Metal Shelf Foot (Autodesk Fusion 360 design; units mm, degrees)
Autodesk Fusion 360 part; units mm, degrees
sketch "Sketch1" plane through (0, 0, 0) normal (0, 0, 1) x (1, 0, 0)
  line L0 (0, 0) -> (46, 0)
  line L1 (46, 0) -> (46, 32)
  line L2 (46, 32) -> (0, 32)
  line L3 (0, 32) -> (0, 0)
  line L4 (-2, 34) -> (48, 34)
  line L5 (48, 34) -> (48, -2)
  line L6 (48, -2) -> (-2, -2)
  line L7 (-2, -2) -> (-2, 34)
  dimension "d1" = 46
  dimension "d2" = 32
  dimension "d3" = 2
  dimension "d4" = 2
  dimension "d5" = 2
  dimension "d6" = 2
  constraint horizontal L0
  constraint vertical L1
  constraint horizontal L2
  constraint vertical L3
  constraint coincident L0.start L3.end
  constraint horizontal L4
  constraint vertical L5
  constraint horizontal L6
  constraint vertical L7
  measures "d1" distance of L0.start L0.end
  measures "d2" distance of L0.start L2.end
  measures "d3" distance of L2 L4
  measures "d4" distance of L3 L7
  measures "d5" distance of L0 L6
  measures "d6" distance of L1 L5
extrude "Extrude1" add sketch "Sketch1" along normal blind 2 contours L0 L1 L2 L3
extrude "Extrude2" add sketch "Sketch1" along normal blind 10
